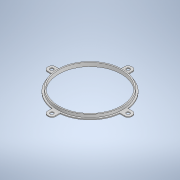
# Autodesk Inventor part: Fan_Part2
Saved by Autodesk Inventor 2020 (Build 240168000, 168)
## iProperties
Created: 2020-05-28
Part Number: Fan_Part2
Material: Generic
Document SubType Name: Modeling
Designer: maple
Density: 1 g/cm^3
Appearance: Default
Author: maple
Autodesk Inventor part; units mm, degrees
ref_plane "YZ Plane" through (0, 0, 0) normal (1, 0, 0) x (0, 1, 0)
ref_plane "XZ Plane" through (0, 0, 0) normal (0, 1, 0) x (-1, 0, 0)
ref_plane "XY Plane" through (0, 0, 0) normal (0, 0, 1) x (1, 0, 0)
sketch "Sketch1" plane through (0, 0, 0) normal (0, 1, 0) x (-1, 0, 0)
  circle A0 centre (0, 0) radius 55
  circle A1 centre (0, 0) radius 60
  line L0 (0, 57.5) -> (7, 57.5)
  line L1 (7, 57.5) -> (-7, 57.5)
  line L2 (7, 57.5) -> (-7, 57.5)
  line L3 (-7, 57.5) -> (-7, 74)
  line L4 (-7, 74) -> (7, 74)
  line L5 (7, 74) -> (7, 57.5)
  line L6 (-74, 7) -> (-57.5, 7)
  line L7 (-74, -7) -> (-74, 7)
  line L8 (-57.5, -7) -> (-74, -7)
  line L9 (-57.5, 7) -> (-57.5, -7)
  line L10 (-7, -74) -> (-7, -57.5)
  line L11 (7, -74) -> (-7, -74)
  line L12 (7, -57.5) -> (7, -74)
  line L13 (-7, -57.5) -> (7, -57.5)
  line L14 (74, -7) -> (57.5, -7)
  line L15 (74, 7) -> (74, -7)
  line L16 (57.5, 7) -> (74, 7)
  line L17 (57.5, -7) -> (57.5, 7)
  point P0 (-7, 59.5903)
  point P1 (-59.5903, 7)
  point P2 (-59.5903, -7)
  point P3 (-7, -59.5903)
  point P4 (7, -59.5903)
  point P5 (59.5903, -7)
  point P6 (59.5903, 7)
  point P7 (7, 59.5903)
  dimension "d0" = 110
  dimension "d1" = 120
  dimension "d2" = 7
  dimension "d3" = 14
  dimension "d7" = 360
  constraints: 36 end point, 3 horizontal, 2 centre point, 2 coincident, 2 parallel, 1 perpendicular, 37 other
  measures "d0" diameter of A0
  measures "d1" diameter of A1
  measures "d2" distance of L0.start L0.end
  measures "d3" distance of L0.end L1.end
extrude "Extrusion1" add sketch "Sketch1" along normal blind 1.5
fillet "Fillet1" radius 6 8 edges at (74, 0.75, -7) (74, 0.75, 7) (7, 0.75, -74) (-7, 0.75, -74) (-74, 0.75, -7) (-74, 0.75, 7) (-7, 0.75, 74) (7, 0.75, 74)
sketch "Sketch2" plane through (0, 1.5, 0) normal (0, 1, 0) x (1, 0, 0)
  line L0 (-1, -74) -> (1, -74) projected
  line L1 (0, -74) -> (0, -67)
  line L2 (74, -1) -> (74, 1) projected
  line L3 (74, 0) -> (67, 0)
  line L4 (1, 74) -> (-1, 74) projected
  line L5 (0, 74) -> (0, 67)
  line L6 (-74, 1) -> (-74, -1) projected
  line L7 (-74, 0) -> (-67, 0)
  point P0 (0, 0)
  dimension "d12" = 7
  dimension "d13" = 7
  dimension "d14" = 7
  dimension "d15" = 7
  constraints: 8 end point, 4 midpoint, 2 horizontal, 2 vertical
  measures "d12" distance of L1.start L1.end
  measures "d13" distance of L3.start L3.end
  measures "d14" distance of L5.start L5.end
  measures "d15" distance of L7.start L7.end
hole "Hole1" at (0, 1.5, 67) at (-67, 1.5, 0) at (0, 1.5, -67) at (67, 1.5, 0) direction (0, -1, 0) diameter 6 end through all
sketch "Sketch3" plane through (0, 1.5, 0) normal (0, 1, 0) x (1, 0, 0)
  circle A0 centre (0, 0) radius 55
  circle A1 centre (0, 0) radius 55 projected
  line L0 (-55, 0) -> (-57, 0)
  circle A2 centre (0, 0) radius 57
  dimension "d23" = 2
  constraints: 2 coincident, 2 end point, 2 horizontal alignment, 1 centre point, 1 horizontal, 3 other
  measures "d23" distance of L0.start L0.end
extrude "Extrusion2" add sketch "Sketch3" along normal blind 5
body "Solid1"
